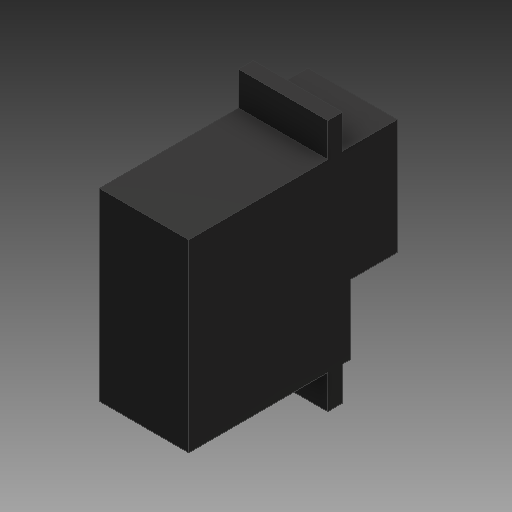
# Autodesk Inventor part: servoMotor
Saved by Autodesk Inventor 2018 (Build 220112000, 112)
## iProperties
Created: 2018-09-18
Part Number: servoMotor
Material: Generic
Document SubType Name: Modeling
Designer: Viraj Shah
Density: 1 g/cm^3
Appearance: Default
Mass: 7.15408 g
Surface Area: 26.5002 cm^2
Volume: 7.15408 cm^3
Author: Viraj Shah
Autodesk Inventor part; units mm, degrees
ref_plane "YZ Plane" through (0, 0, 0) normal (1, 0, 0) x (0, 1, 0)
ref_plane "XZ Plane" through (0, 0, 0) normal (0, 1, 0) x (-1, 0, 0)
ref_plane "XY Plane" through (0, 0, 0) normal (0, 0, 1) x (1, 0, 0)
sketch "Sketch1" plane through (0, 0, 0) normal (1, 0, 0) x (0, 1, 0)
  line L0 (10.5, 12) -> (-10.5, 12)
  line L1 (-10.5, 12) -> (-10.5, -12)
  line L2 (-10.5, -12) -> (10.5, -12)
  line L3 (10.5, -12) -> (10.5, 12)
  line L4 (10.5, 12) -> (-10.5, -12) construction
  line L5 (-10.5, 12) -> (10.5, -12) construction
  point P0 (0, 0)
  dimension "d0" = 21
  dimension "d1" = 24
  constraints: 12 end point, 2 midpoint, 2 parallel, 1 horizontal, 1 perpendicular
  measures "d0" distance of L2.end L1.end
  measures "d1" distance of L2.end L0.start
extrude "Extrusion1" add sketch "Sketch1" along normal mid plane 11.6
sketch "Sketch2" plane through (5.8, 0, 0) normal (1, 0, 0) x (0, 0, -1)
  line L0 (-12, 9.5) -> (-16.4, 9.5)
  line L1 (-16.4, 9.5) -> (-16.4, 7.58)
  line L2 (-16.4, 7.58) -> (-12, 7.58)
  line L3 (-12, 7.58) -> (-12, 9.5)
  line L4 (-12, -10.5) -> (12, -10.5) projected
  line L5 (0, -10.5) -> (0, 10.5)
  line L6 (12, 9.5) -> (16.4, 9.5)
  line L7 (16.4, 9.5) -> (16.4, 7.58)
  line L8 (16.4, 7.58) -> (12, 7.58)
  line L9 (12, 7.58) -> (12, 9.5)
  line L10 (-12, 9.5) -> (-13.7444, 9.5)
  point P0 (0, 0)
  point P1 (-12, 10.5)
  dimension "d4" = 4.4
  dimension "d5" = 1.92
  dimension "d8" = 1
  constraints: 21 end point, 4 symmetric about line, 2 parallel, 2 perpendicular, 1 horizontal, 1 midpoint, 1 vertical
  measures "d4" distance of L2.end L1.end
  measures "d5" distance of L1.end L0.end
  measures "d8" distance of point (-12, 10.5) L0.start
extrude "Extrusion2" add sketch "Sketch2" against normal up to surface (11.6 mm away)
sketch "Sketch3" plane through (5.8, 0, 0) normal (1, 0, 0) x (0, 0, -1)
  line L0 (-12, 10.5) -> (3, 10.5)
  line L1 (3, 10.5) -> (3, 16.6)
  line L2 (3, 16.6) -> (-12, 16.6)
  line L3 (-12, 16.6) -> (-12, 10.5)
  line L4 (12, 10.5) -> (-12, 10.5) projected
  point P0 (0, 0)
  dimension "d9" = 15
  dimension "d10" = 6.1
  constraints: 8 end point, 2 parallel, 1 horizontal, 1 perpendicular
  measures "d9" distance of L2.end L1.end
  measures "d10" distance of L0.start L2.end
extrude "Extrusion3" add sketch "Sketch3" against normal up to surface (11.6 mm away)
sketch "Sketch4" plane through (5.8, 16.6, 12) normal (0, 1, 0) x (1, 0, 0)
  circle A0 centre (-5.8, 6.9504) radius 2.829
  point P0 (-5.8, 12)
  constraints: 1 centre point
extrude "Extrusion4" add sketch "Sketch4" along normal blind 2
body "Solid1"
